Autodesk Fusion 360 part; units mm, degrees
(part 2 of 2)
sketch "Sketch21" plane through (0, 0, 6.5) normal (0, 0, 1) x (-1, 0, 0)
  line L0 (-17.15, -12.5) -> (-13.9, -12.5)
  line L1 (-13.9, -12.5) -> (-13.9, -16.5)
  line L2 (-13.9, -16.5) -> (-17.15, -16.5)
  line L3 (-17.15, -16.5) -> (-17.15, -12.5)
  line L4 (-52.0582, -15.8447) -> (-53.0435, -16.5507)
  line L5 (-53.0435, -16.5507) -> (-52.0582, -17.32)
  line L6 (-52.0582, -17.32) -> (-52.3471, -17.6537)
  line L7 (-52.3471, -17.6537) -> (-53.2, -17)
  line L8 (-53.2, -17) -> (-53.2, -19.1)
  line L9 (-53.2, -19.1) -> (-53.5525, -19.2486)
  line L10 (-53.5525, -19.2486) -> (-55.3569, -17.8655)
  line L11 (-55.3569, -17.8655) -> (-55.3569, -17.6445)
  line L12 (-55.3569, -17.6445) -> (-53.8076, -16.5343)
  line L13 (-53.8076, -16.5343) -> (-55.2956, -15.447)
  line L14 (-55.2956, -15.447) -> (-55.2956, -15.2)
  line L15 (-55.2956, -15.2) -> (-53.5478, -13.8892)
  line L16 (-53.5478, -13.8892) -> (-53.3624, -13.8892)
  line L17 (-53.3624, -13.8892) -> (-53.1862, -14.0561)
  line L18 (-53.1862, -14.0561) -> (-53.1862, -16.0889)
  line L19 (-53.1862, -16.0889) -> (-52.3253, -15.472)
  line L20 (-52.3253, -15.472) -> (-52.0582, -15.8447)
  line L21 (-15.85, -17.05) -> (-15.85, -21.05)
  line L22 (-15.85, -21.05) -> (-19.85, -21.05)
  line L23 (-19.85, -21.05) -> (-19.85, -17.05)
  line L24 (-19.85, -17.05) -> (-15.85, -17.05)
  line L25 (-28.1, -12) -> (-28.1, -6.3)
  line L26 (-28.1, -6.3) -> (-14, -6.3)
  line L27 (-14, -6.3) -> (-14, -12)
  line L28 (-14, -12) -> (-28.1, -12)
  line L29 (-57.9, -11.55) -> (-57.9, -8.9)
  arc A0 (-57.4639, -4.5) -> (-57.9, -8.9) centre (-59.7, -6.5) ccw
  line L30 (-57.4639, -4.5) -> (-46.1, -4.5)
  line L31 (-46.1, -4.5) -> (-46.1, -11.55)
  line L32 (-46.1, -11.55) -> (-57.9, -11.55)
  line L33 (-16.8084, -5.642) -> (-16.8084, -3.2045)
  line L34 (-16.8084, -3.2045) -> (-16.4431, -3.2045)
  line L35 (-16.4431, -3.2045) -> (-16.4431, -6.0678)
  line L36 (-16.4431, -6.0678) -> (-17.0134, -6.0678)
  line L37 (-17.0134, -6.0678) -> (-17.6912, -4.0404)
  spline S0 degree 3 poles (-17.6912, -4.0404) (-17.7185, -3.958) (-17.7651, -3.817) (-17.8095, -3.6754) (-17.8279, -3.6166) knots 0 0 0 0 0.026049 0.044534 0.044534 0.044534 0.044534
  spline S1 degree 3 poles (-17.8279, -3.6166) (-17.8486, -3.6809) (-17.8979, -3.8344) (-17.95, -3.987) (-17.9802, -4.0756) knots 0 0 0 0 0.020274 0.048362 0.048362 0.048362 0.048362
  line L38 (-17.9802, -4.0756) -> (-18.6658, -6.0678)
  line L39 (-18.6658, -6.0678) -> (-19.1756, -6.0678)
  line L40 (-19.1756, -6.0678) -> (-19.1756, -3.2045)
  line L41 (-19.1756, -3.2045) -> (-18.8103, -3.2045)
  line L42 (-18.8103, -3.2045) -> (-18.8103, -5.601)
  line L43 (-18.8103, -5.601) -> (-17.9783, -3.2045)
  line L44 (-17.9783, -3.2045) -> (-17.6365, -3.2045)
  line L45 (-17.6365, -3.2045) -> (-16.8084, -5.642)
  spline S2 degree 3 poles (-27.6951, -3.1556) (-27.5655, -3.1667) (-27.3128, -3.1883) (-27.1326, -3.3659) (-27.0447, -3.4525) knots 0 0 0 0 0.037701 0.073534 0.073534 0.073534 0.073534
  spline S3 degree 3 poles (-27.0447, -3.4525) (-26.9626, -3.606) (-26.7692, -3.9674) (-26.7643, -4.3795) (-26.7615, -4.6166) knots 0 0 0 0 0.051552 0.121345 0.121345 0.121345 0.121345
  spline S4 degree 3 poles (-26.7615, -4.6166) (-26.7636, -4.7702) (-26.7673, -5.047) (-26.8356, -5.3148) (-26.866, -5.434) knots 0 0 0 0 0.0459 0.082658 0.082658 0.082658 0.082658
  spline S5 degree 3 poles (-26.866, -5.434) (-26.903, -5.5295) (-26.9732, -5.7107) (-27.1113, -5.8471) (-27.1765, -5.9115) knots 0 0 0 0 0.030338 0.057541 0.057541 0.057541 0.057541
  spline S6 degree 3 poles (-27.1765, -5.9115) (-27.2518, -5.9605) (-27.4092, -6.0629) (-27.597, -6.0738) (-27.6951, -6.0795) knots 0 0 0 0 0.026458 0.055354 0.055354 0.055354 0.055354
  spline S7 degree 3 poles (-27.6951, -6.0795) (-27.7683, -6.0763) (-27.9088, -6.0701) (-28.0376, -6.0137) (-28.0994, -5.9867) knots 0 0 0 0 0.021755 0.0418 0.0418 0.0418 0.0418
  spline S8 degree 3 poles (-28.0994, -5.9867) (-28.1551, -5.9519) (-28.2681, -5.8814) (-28.3466, -5.7737) (-28.3865, -5.7191) knots 0 0 0 0 0.019498 0.039572 0.039572 0.039572 0.039572
  spline S9 degree 3 poles (-28.3865, -5.7191) (-28.4227, -5.6556) (-28.4995, -5.5211) (-28.5419, -5.372) (-28.5642, -5.2933) knots 0 0 0 0 0.021862 0.046289 0.046289 0.046289 0.046289
  spline S10 degree 3 poles (-28.5642, -5.2933) (-28.583, -5.1954) (-28.6257, -4.972) (-28.6276, -4.7444) (-28.6287, -4.6166) knots 0 0 0 0 0.029862 0.068104 0.068104 0.068104 0.068104
  spline S11 degree 3 poles (-28.6287, -4.6166) (-28.6266, -4.4639) (-28.6228, -4.1886) (-28.5553, -3.9219) (-28.5252, -3.8031) knots 0 0 0 0 0.045606 0.082253 0.082253 0.082253 0.082253
  spline S12 degree 3 poles (-28.5252, -3.8031) (-28.4884, -3.7075) (-28.4186, -3.526) (-28.2808, -3.3893) (-28.2156, -3.3246) knots 0 0 0 0 0.030329 0.05757 0.05757 0.05757 0.05757
  spline S13 degree 3 poles (-28.2156, -3.3246) (-28.1402, -3.2753) (-27.9823, -3.1722) (-27.7937, -3.1613) (-27.6951, -3.1556) knots 0 0 0 0 0.026536 0.05558 0.05558 0.05558 0.05558
  spline S14 degree 3 poles (-24.533, -4.0326) (-24.5377, -4.1203) (-24.5468, -4.2881) (-24.6333, -4.4318) (-24.6746, -4.5004) knots 0 0 0 0 0.025902 0.04954 0.04954 0.04954 0.04954
  spline S15 degree 3 poles (-24.6746, -4.5004) (-24.7283, -4.5586) (-24.8399, -4.6795) (-24.9966, -4.7307) (-25.0779, -4.7572) knots 0 0 0 0 0.023359 0.04853 0.04853 0.04853 0.04853
  spline S16 degree 3 poles (-25.0779, -4.7572) (-25.0111, -4.7849) (-24.8856, -4.8369) (-24.7957, -4.9383) (-24.7537, -4.9857) knots 0 0 0 0 0.021379 0.040128 0.040128 0.040128 0.040128
  spline S17 degree 3 poles (-24.7537, -4.9857) (-24.7229, -5.0388) (-24.6592, -5.1486) (-24.652, -5.2755) (-24.6482, -5.3412) knots 0 0 0 0 0.018126 0.037544 0.037544 0.037544 0.037544
  spline S18 degree 3 poles (-24.6482, -5.3412) (-24.6575, -5.4411) (-24.6759, -5.6404) (-24.8073, -5.7913) (-24.8728, -5.8666) knots 0 0 0 0 0.029303 0.058444 0.058444 0.058444 0.058444
  spline S19 degree 3 poles (-24.8728, -5.8666) (-24.9568, -5.9286) (-25.134, -6.0595) (-25.3545, -6.0726) (-25.4705, -6.0795) knots 0 0 0 0 0.030658 0.064671 0.064671 0.064671 0.064671
  spline S20 degree 3 poles (-25.4705, -6.0795) (-25.5873, -6.0723) (-25.8104, -6.0585) (-25.989, -5.9252) (-26.074, -5.8617) knots 0 0 0 0 0.034273 0.065414 0.065414 0.065414 0.065414
  spline S21 degree 3 poles (-26.074, -5.8617) (-26.1406, -5.7853) (-26.2736, -5.633) (-26.2929, -5.4317) (-26.3025, -5.3314) knots 0 0 0 0 0.02961 0.059051 0.059051 0.059051 0.059051
  spline S22 degree 3 poles (-26.3025, -5.3314) (-26.2986, -5.2679) (-26.2911, -5.144) (-26.2285, -5.0369) (-26.198, -4.9847) knots 0 0 0 0 0.01881 0.036662 0.036662 0.036662 0.036662
  spline S23 degree 3 poles (-26.198, -4.9847) (-26.1567, -4.9377) (-26.0687, -4.8375) (-25.9458, -4.785) (-25.8806, -4.7572) knots 0 0 0 0 0.018541 0.039496 0.039496 0.039496 0.039496
  spline S24 degree 3 poles (-25.8806, -4.7572) (-25.9622, -4.7257) (-26.1184, -4.6652) (-26.2291, -4.5398) (-26.282, -4.4799) knots 0 0 0 0 0.025791 0.049427 0.049427 0.049427 0.049427
  spline S25 degree 3 poles (-26.282, -4.4799) (-26.3222, -4.4116) (-26.4051, -4.2707) (-26.4147, -4.1072) (-26.4197, -4.0228) knots 0 0 0 0 0.023398 0.048344 0.048344 0.048344 0.048344
  spline S26 degree 3 poles (-26.4197, -4.0228) (-26.4091, -3.9055) (-26.388, -3.6722) (-26.2357, -3.4942) (-26.1599, -3.4056) knots 0 0 0 0 0.034407 0.068461 0.068461 0.068461 0.068461
  spline S27 degree 3 poles (-26.1599, -3.4056) (-26.0636, -3.3328) (-25.8618, -3.1801) (-25.6086, -3.164) (-25.4763, -3.1556) knots 0 0 0 0 0.035444 0.074232 0.074232 0.074232 0.074232
  spline S28 degree 3 poles (-25.4763, -3.1556) (-25.344, -3.1641) (-25.0907, -3.1803) (-24.8891, -3.3335) (-24.7927, -3.4066) knots 0 0 0 0 0.038792 0.074275 0.074275 0.074275 0.074275
  spline S29 degree 3 poles (-24.7927, -3.4066) (-24.717, -3.4961) (-24.5638, -3.677) (-24.5433, -3.9132) (-24.533, -4.0326) knots 0 0 0 0 0.034274 0.069281 0.069281 0.069281 0.069281
  line L46 (-61.2402, -13.1835) -> (-61.2402, -11.8827)
  line L47 (-61.2402, -11.8827) -> (-60.8613, -11.8827)
  line L48 (-60.8613, -11.8827) -> (-60.8613, -14.746)
  line L49 (-60.8613, -14.746) -> (-62.793, -14.746)
  line L50 (-62.793, -14.746) -> (-62.793, -14.4081)
  line L51 (-62.793, -14.4081) -> (-61.2402, -14.4081)
  line L52 (-61.2402, -14.4081) -> (-61.2402, -13.5213)
  line L53 (-61.2402, -13.5213) -> (-62.584, -13.5213)
  line L54 (-62.584, -13.5213) -> (-62.584, -13.1835)
  line L55 (-62.584, -13.1835) -> (-61.2402, -13.1835)
  line L56 (-50.1317, -14.1836) -> (-50.1317, -11.9336)
  line L57 (-50.1317, -11.9336) -> (-49.7684, -11.9336)
  line L58 (-49.7684, -11.9336) -> (-49.7684, -14.7969)
  line L59 (-49.7684, -14.7969) -> (-50.1571, -14.7969)
  line L60 (-50.1571, -14.7969) -> (-51.661, -12.5488)
  line L61 (-51.661, -12.5488) -> (-51.661, -14.7969)
  line L62 (-51.661, -14.7969) -> (-52.0243, -14.7969)
  line L63 (-52.0243, -14.7969) -> (-52.0243, -11.9336)
  line L64 (-52.0243, -11.9336) -> (-51.6356, -11.9336)
  line L65 (-51.6356, -11.9336) -> (-50.1317, -14.1836)
  spline S30 degree 3 poles (-47.1923, -12.0801) (-47.0925, -12.1512) (-46.8928, -12.2937) (-46.7709, -12.5067) (-46.7098, -12.6133) knots 0 0 0 0 0.03628 0.072668 0.072668 0.072668 0.072668
  spline S31 degree 3 poles (-46.7098, -12.6133) (-46.662, -12.7276) (-46.5662, -12.9565) (-46.5526, -13.2042) (-46.5458, -13.3281) knots 0 0 0 0 0.036879 0.073826 0.073826 0.073826 0.073826
  spline S32 degree 3 poles (-46.5458, -13.3281) (-46.5569, -13.5474) (-46.5776, -13.9578) (-46.8171, -14.2898) (-46.9286, -14.4444) knots 0 0 0 0 0.064266 0.120259 0.120259 0.120259 0.120259
  spline S33 degree 3 poles (-46.9286, -14.4444) (-47.0678, -14.562) (-47.3531, -14.803) (-47.726, -14.8325) (-47.9169, -14.8477) knots 0 0 0 0 0.053269 0.109167 0.109167 0.109167 0.109167
  spline S34 degree 3 poles (-47.9169, -14.8477) (-48.0448, -14.8404) (-48.2961, -14.826) (-48.5212, -14.7135) (-48.6317, -14.6582) knots 0 0 0 0 0.037992 0.074647 0.074647 0.074647 0.074647
  spline S35 degree 3 poles (-48.6317, -14.6582) (-48.7317, -14.5886) (-48.9326, -14.4485) (-49.0554, -14.2365) (-49.1171, -14.1299) knots 0 0 0 0 0.036074 0.072525 0.072525 0.072525 0.072525
  spline S36 degree 3 poles (-49.1171, -14.1299) (-49.1658, -14.0109) (-49.2665, -13.7647) (-49.2781, -13.4988) (-49.2841, -13.3613) knots 0 0 0 0 0.038265 0.079177 0.079177 0.079177 0.079177
  spline S37 degree 3 poles (-49.2841, -13.3613) (-49.2777, -13.2219) (-49.2654, -12.9515) (-49.1595, -12.7026) (-49.1083, -12.582) knots 0 0 0 0 0.041493 0.080461 0.080461 0.080461 0.080461
  spline S38 degree 3 poles (-49.1083, -12.582) (-49.0443, -12.4748) (-48.918, -12.2632) (-48.7119, -12.1282) (-48.6102, -12.0615) knots 0 0 0 0 0.036922 0.072885 0.072885 0.072885 0.072885
  spline S39 degree 3 poles (-48.6102, -12.0615) (-48.5005, -12.01) (-48.28, -11.9065) (-48.0369, -11.892) (-47.9149, -11.8848) knots 0 0 0 0 0.036024 0.072329 0.072329 0.072329 0.072329
  spline S40 degree 3 poles (-47.9149, -11.8848) (-47.7849, -11.8922) (-47.5302, -11.9068) (-47.3033, -12.0231) (-47.1923, -12.0801) knots 0 0 0 0 0.038591 0.075598 0.075598 0.075598 0.075598
  line L66 (-58.7969, -13.1835) -> (-58.7969, -11.8827)
  line L67 (-58.7969, -11.8827) -> (-58.418, -11.8827)
  line L68 (-58.418, -11.8827) -> (-58.418, -14.746)
  line L69 (-58.418, -14.746) -> (-60.3496, -14.746)
  line L70 (-60.3496, -14.746) -> (-60.3496, -14.4081)
  line L71 (-60.3496, -14.4081) -> (-58.7969, -14.4081)
  line L72 (-58.7969, -14.4081) -> (-58.7969, -13.5213)
  line L73 (-58.7969, -13.5213) -> (-60.1406, -13.5213)
  line L74 (-60.1406, -13.5213) -> (-60.1406, -13.1835)
  line L75 (-60.1406, -13.1835) -> (-58.7969, -13.1835)
  spline S41 degree 3 poles (-55.8183, -12.0292) (-55.7186, -12.1003) (-55.5188, -12.2428) (-55.397, -12.4557) (-55.3359, -12.5624) knots 0 0 0 0 0.03628 0.072668 0.072668 0.072668 0.072668
  spline S42 degree 3 poles (-55.3359, -12.5624) (-55.2881, -12.6767) (-55.1923, -12.9055) (-55.1787, -13.1532) (-55.1719, -13.2772) knots 0 0 0 0 0.036879 0.073826 0.073826 0.073826 0.073826
  spline S43 degree 3 poles (-55.1719, -13.2772) (-55.1829, -13.4965) (-55.2037, -13.9068) (-55.4432, -14.2388) (-55.5547, -14.3934) knots 0 0 0 0 0.064266 0.120259 0.120259 0.120259 0.120259
  spline S44 degree 3 poles (-55.5547, -14.3934) (-55.6939, -14.511) (-55.9792, -14.7521) (-56.352, -14.7816) (-56.543, -14.7967) knots 0 0 0 0 0.053269 0.109167 0.109167 0.109167 0.109167
  spline S45 degree 3 poles (-56.543, -14.7967) (-56.6709, -14.7894) (-56.9222, -14.7751) (-57.1473, -14.6625) (-57.2578, -14.6073) knots 0 0 0 0 0.037992 0.074647 0.074647 0.074647 0.074647
  spline S46 degree 3 poles (-57.2578, -14.6073) (-57.3578, -14.5376) (-57.5587, -14.3975) (-57.6815, -14.1855) (-57.7431, -14.079) knots 0 0 0 0 0.036074 0.072525 0.072525 0.072525 0.072525
  spline S47 degree 3 poles (-57.7431, -14.079) (-57.7918, -13.96) (-57.8926, -13.7138) (-57.9042, -13.4478) (-57.9101, -13.3104) knots 0 0 0 0 0.038265 0.079177 0.079177 0.079177 0.079177
  spline S48 degree 3 poles (-57.9101, -13.3104) (-57.9038, -13.171) (-57.8914, -12.9006) (-57.7856, -12.6517) (-57.7344, -12.5311) knots 0 0 0 0 0.041493 0.080461 0.080461 0.080461 0.080461
  spline S49 degree 3 poles (-57.7344, -12.5311) (-57.6704, -12.4239) (-57.5441, -12.2122) (-57.338, -12.0772) (-57.2363, -12.0106) knots 0 0 0 0 0.036922 0.072885 0.072885 0.072885 0.072885
  spline S50 degree 3 poles (-57.2363, -12.0106) (-57.1265, -11.959) (-56.9061, -11.8555) (-56.663, -11.8411) (-56.541, -11.8338) knots 0 0 0 0 0.036024 0.072329 0.072329 0.072329 0.072329
  spline S51 degree 3 poles (-56.541, -11.8338) (-56.411, -11.8413) (-56.1563, -11.8558) (-55.9294, -11.9722) (-55.8183, -12.0292) knots 0 0 0 0 0.038591 0.075598 0.075598 0.075598 0.075598
  spline S52 degree 3 poles (-22.9041, -3.7328) (-22.8758, -3.7018) (-22.8214, -3.6422) (-22.777, -3.5748) (-22.7556, -3.5424) knots 0 0 0 0 0.012549 0.024178 0.024178 0.024178 0.024178
  line L76 (-22.7556, -3.5424) -> (-24.1599, -3.5424)
  line L77 (-24.1599, -3.5424) -> (-24.1599, -3.2045)
  line L78 (-24.1599, -3.2045) -> (-22.2674, -3.2045)
  spline S53 degree 3 poles (-22.2674, -3.2045) (-22.2681, -3.2463) (-22.2695, -3.3298) (-22.2954, -3.4091) (-22.3084, -3.4486) knots 0 0 0 0 0.012479 0.024881 0.024881 0.024881 0.024881
  spline S54 degree 3 poles (-22.3084, -3.4486) (-22.3372, -3.5141) (-22.3975, -3.6512) (-22.491, -3.7683) (-22.5398, -3.8295) knots 0 0 0 0 0.021368 0.044735 0.044735 0.044735 0.044735
  spline S55 degree 3 poles (-22.5398, -3.8295) (-22.6034, -3.8982) (-22.7469, -4.0531) (-22.9094, -4.188) (-22.9998, -4.2631) knots 0 0 0 0 0.028058 0.063271 0.063271 0.063271 0.063271
  spline S56 degree 3 poles (-22.9998, -4.2631) (-23.1342, -4.3733) (-23.3607, -4.5589) (-23.5526, -4.7798) (-23.6306, -4.8695) knots 0 0 0 0 0.052022 0.087641 0.087641 0.087641 0.087641
  spline S57 degree 3 poles (-23.6306, -4.8695) (-23.6784, -4.9395) (-23.7661, -5.0682) (-23.7857, -5.2222) (-23.7947, -5.2924) knots 0 0 0 0 0.024992 0.04593 0.04593 0.04593 0.04593
  spline S58 degree 3 poles (-23.7947, -5.2924) (-23.7885, -5.3592) (-23.7762, -5.4927) (-23.6889, -5.5942) (-23.6453, -5.6449) knots 0 0 0 0 0.019622 0.039148 0.039148 0.039148 0.039148
  spline S59 degree 3 poles (-23.6453, -5.6449) (-23.5902, -5.6868) (-23.4752, -5.774) (-23.3308, -5.7835) (-23.2556, -5.7885) knots 0 0 0 0 0.020302 0.042349 0.042349 0.042349 0.042349
  spline S60 degree 3 poles (-23.2556, -5.7885) (-23.1765, -5.7834) (-23.0253, -5.7736) (-22.9062, -5.6805) (-22.8494, -5.6361) knots 0 0 0 0 0.023167 0.044296 0.044296 0.044296 0.044296
  spline S61 degree 3 poles (-22.8494, -5.6361) (-22.8049, -5.5779) (-22.71, -5.4538) (-22.7003, -5.2974) (-22.6951, -5.2142) knots 0 0 0 0 0.021485 0.045832 0.045832 0.045832 0.045832
  line L79 (-22.6951, -5.2142) -> (-22.3338, -5.2513)
  spline S62 degree 3 poles (-22.3338, -5.2513) (-22.3518, -5.3754) (-22.3857, -5.6086) (-22.5406, -5.785) (-22.6131, -5.8676) knots 0 0 0 0 0.0367 0.068958 0.068958 0.068958 0.068958
  spline S63 degree 3 poles (-22.6131, -5.8676) (-22.7047, -5.9293) (-22.9006, -6.0614) (-23.1374, -6.0732) (-23.2634, -6.0795) knots 0 0 0 0 0.032518 0.069569 0.069569 0.069569 0.069569
  spline S64 degree 3 poles (-23.2634, -6.0795) (-23.3909, -6.0725) (-23.6312, -6.0593) (-23.8248, -5.9175) (-23.9158, -5.851) knots 0 0 0 0 0.037354 0.070456 0.070456 0.070456 0.070456
  spline S65 degree 3 poles (-23.9158, -5.851) (-23.9859, -5.7699) (-24.1267, -5.607) (-24.1462, -5.3924) (-24.156, -5.2845) knots 0 0 0 0 0.031293 0.062923 0.062923 0.062923 0.062923
  spline S66 degree 3 poles (-24.156, -5.2845) (-24.153, -5.2272) (-24.1467, -5.111) (-24.1062, -5.0019) (-24.0857, -4.9467) knots 0 0 0 0 0.017131 0.03469 0.03469 0.03469 0.03469
  spline S67 degree 3 poles (-24.0857, -4.9467) (-24.0566, -4.8885) (-23.9933, -4.7624) (-23.9017, -4.655) (-23.8523, -4.597) knots 0 0 0 0 0.019438 0.042172 0.042172 0.042172 0.042172
  spline S68 degree 3 poles (-23.8523, -4.597) (-23.7809, -4.5234) (-23.609, -4.3462) (-23.4205, -4.1865) (-23.3103, -4.0931) knots 0 0 0 0 0.030746 0.074043 0.074043 0.074043 0.074043
  spline S69 degree 3 poles (-23.3103, -4.0931) (-23.2227, -4.02) (-23.0836, -3.904) (-22.9525, -3.779) (-22.9041, -3.7328) knots 0 0 0 0 0.034229 0.054317 0.054317 0.054317 0.054317
  line L80 (-20.1658, -4.3685) -> (-20.1658, -3.2045)
  line L81 (-20.1658, -3.2045) -> (-19.7869, -3.2045)
  line L82 (-19.7869, -3.2045) -> (-19.7869, -6.0678)
  line L83 (-19.7869, -6.0678) -> (-20.867, -6.0678)
  spline S70 degree 3 poles (-20.867, -6.0678) (-20.9509, -6.0675) (-21.0967, -6.067) (-21.2412, -6.0483) (-21.3025, -6.0404) knots 0 0 0 0 0.025156 0.043678 0.043678 0.043678 0.043678
  spline S71 degree 3 poles (-21.3025, -6.0404) (-21.3685, -6.027) (-21.4938, -6.0016) (-21.6039, -5.9371) (-21.656, -5.9066) knots 0 0 0 0 0.020045 0.038029 0.038029 0.038029 0.038029
  spline S72 degree 3 poles (-21.656, -5.9066) (-21.7017, -5.8695) (-21.7963, -5.7925) (-21.8551, -5.6856) (-21.8855, -5.6303) knots 0 0 0 0 0.017485 0.036225 0.036225 0.036225 0.036225
  spline S73 degree 3 poles (-21.8855, -5.6303) (-21.9109, -5.5689) (-21.9625, -5.4438) (-21.9691, -5.3085) (-21.9724, -5.2396) knots 0 0 0 0 0.019759 0.040284 0.040284 0.040284 0.040284
  spline S74 degree 3 poles (-21.9724, -5.2396) (-21.9634, -5.1233) (-21.9457, -4.8946) (-21.8078, -4.7115) (-21.74, -4.6215) knots 0 0 0 0 0.034213 0.067281 0.067281 0.067281 0.067281
  spline S75 degree 3 poles (-21.74, -4.6215) (-21.6347, -4.5481) (-21.3849, -4.3742) (-21.0778, -4.3706) (-20.9002, -4.3685) knots 0 0 0 0 0.037732 0.089487 0.089487 0.089487 0.089487
  line L84 (-20.9002, -4.3685) -> (-20.1658, -4.3685)
  spline S76 degree 3 poles (-15.325, -3.2523) (-15.2553, -3.2384) (-15.1029, -3.2079) (-14.9474, -3.2057) (-14.8631, -3.2045) knots 0 0 0 0 0.021277 0.046525 0.046525 0.046525 0.046525
  line L85 (-14.8631, -3.2045) -> (-13.7713, -3.2045)
  line L86 (-13.7713, -3.2045) -> (-13.7713, -6.0678)
  line L87 (-13.7713, -6.0678) -> (-14.8455, -6.0678)
  spline S77 degree 3 poles (-14.8455, -6.0678) (-14.945, -6.0659) (-15.125, -6.0626) (-15.2956, -6.0061) (-15.3718, -5.9808) knots 0 0 0 0 0.029645 0.05362 0.05362 0.05362 0.05362
  spline S78 degree 3 poles (-15.3718, -5.9808) (-15.4343, -5.9481) (-15.5585, -5.8829) (-15.6412, -5.7696) (-15.6824, -5.7133) knots 0 0 0 0 0.020838 0.041482 0.041482 0.041482 0.041482
  spline S79 degree 3 poles (-15.6824, -5.7133) (-15.7151, -5.653) (-15.7794, -5.5349) (-15.7897, -5.401) (-15.7947, -5.3353) knots 0 0 0 0 0.02031 0.039825 0.039825 0.039825 0.039825
  spline S80 degree 3 poles (-15.7947, -5.3353) (-15.7904, -5.2748) (-15.7817, -5.1525) (-15.7241, -5.0443) (-15.6951, -4.9896) knots 0 0 0 0 0.017995 0.036334 0.036334 0.036334 0.036334
  spline S81 degree 3 poles (-15.6951, -4.9896) (-15.6563, -4.9375) (-15.5752, -4.8286) (-15.4563, -4.7624) (-15.3943, -4.7279) knots 0 0 0 0 0.019257 0.040275 0.040275 0.040275 0.040275
  spline S82 degree 3 poles (-15.3943, -4.7279) (-15.4748, -4.6995) (-15.6291, -4.6449) (-15.7404, -4.5253) (-15.7937, -4.4681) knots 0 0 0 0 0.025178 0.048277 0.048277 0.048277 0.048277
  spline S83 degree 3 poles (-15.7937, -4.4681) (-15.8344, -4.4033) (-15.9177, -4.2707) (-15.9281, -4.1144) (-15.9334, -4.0345) knots 0 0 0 0 0.022594 0.046193 0.046193 0.046193 0.046193
  spline S84 degree 3 poles (-15.9334, -4.0345) (-15.93, -3.969) (-15.9233, -3.8394) (-15.8732, -3.7197) (-15.8484, -3.6605) knots 0 0 0 0 0.019525 0.038613 0.038613 0.038613 0.038613
  spline S85 degree 3 poles (-15.8484, -3.6605) (-15.8197, -3.6072) (-15.7652, -3.506) (-15.6791, -3.4299) (-15.6384, -3.3939) knots 0 0 0 0 0.018014 0.034173 0.034173 0.034173 0.034173
  spline S86 degree 3 poles (-15.6384, -3.3939) (-15.5925, -3.3642) (-15.4953, -3.3012) (-15.3838, -3.2692) (-15.325, -3.2523) knots 0 0 0 0 0.016314 0.034565 0.034565 0.034565 0.034565
  line L88 (-44, -14.3465) -> (-44, -8.4135)
  arc A1 (-44, -14.3465) -> (-44, -8.4135) centre (-38.9, -11.38) ccw
  circle A2 centre (-9.7, -18.5) radius 3
  circle A3 centre (-59.7, -18.5) radius 3
  line L89 (-3, -22) -> (-3, -3)
  line L90 (-3, -3) -> (-66.4, -3)
  line L91 (-66.4, -3) -> (-66.4, -22)
  line L92 (-66.4, -22) -> (-3, -22)
  circle A4 centre (-9.7, -6.5) radius 3
  circle A5 centre (-38.9, -11.38) radius 7.9
  line L93 (-56.4, -6) -> (-47.6, -6)
  line L94 (-47.6, -6) -> (-47.6, -10.05)
  line L95 (-47.6, -10.05) -> (-56.4, -10.05)
  line L96 (-56.4, -10.05) -> (-56.4, -6)
  line L97 (-57.9, -11.55) -> (-46.1, -11.55)
  line L98 (-46.1, -11.55) -> (-46.1, -4.5)
  line L99 (-46.1, -4.5) -> (-57.9, -4.5)
  line L100 (-57.9, -4.5) -> (-57.9, -11.55)
  dimension "d162" = 15.8
  constraint concentric A1 A5
  measures "d162" diameter of A5
extrude "Extrude25" cut sketch "Sketch21" against normal up to surface (4.5 mm away) contours L31 L32 A5 L97 L98 bodies 1
sketch "Sketch13" plane through (0, 0, 2) normal (0, 0, 1) x (-1, 0, 0)
  spline S0 degree 5 poles (-13, -21) (-12.9646, -20.9538) (-12.9119, -20.8347) (-12.8858, -20.5685) (-12.9434, -20.0302) (-13.1125, -19.1087) (-13.3117, -18.0419) (-13.4771, -16.9472) (-13.5596, -15.9266) (-13.5404, -15.0289) (-13.4343, -14.2416) (-13.2755, -13.5173) (-13.1092, -12.792) (-12.9804, -12.0068) (-12.9236, -11.1274) (-12.9529, -10.1651) (-13.0679, -9.1622) (-13.2599, -8.1778) (-13.5174, -7.2746) (-13.8326, -6.5044) (-14.2066, -5.8947) (-14.6566, -5.4341) (-15.207, -5.0857) (-15.8804, -4.8045) (-16.6894, -4.551) (-17.6257, -4.3096) (-18.6571, -4.0958) (-19.7378, -3.9412) (-20.8164, -3.8828) (-21.8447, -3.951) (-22.787, -4.1576) (-23.627, -4.4852) (-24.3799, -4.8712) (-25.083, -5.2256) (-25.7801, -5.4598) (-26.5066, -5.5143) (-27.2774, -5.3814) (-28.0674, -5.1423) (-28.8173, -4.9489) (-29.4603, -4.9571) (-29.9425, -5.2749) (-30.2462, -5.903) (-30.411, -6.6831) (-30.5087, -7.3832) (-30.6209, -7.7798) (-30.8155, -7.7387) (-31.1224, -7.3008) (-31.5439, -6.6155) (-32.0647, -5.8711) (-32.6632, -5.2226) (-33.3205, -4.7328) (-34.0208, -4.4037) (-34.7521, -4.1964) (-35.5076, -4.0563) (-36.2858, -3.9352) (-37.0922, -3.816) (-37.9338, -3.7038) (-38.8151, -3.6163) (-39.7321, -3.5743) (-40.6685, -3.5925) (-41.5893, -3.6694) (-42.4405, -3.7812) (-43.1695, -3.8957) (-43.7428, -3.9816) (-44.162, -4.0192) (-44.4879, -4.0139) (-44.8361, -3.9961) (-45.3251, -3.9983) (-46.0262, -4.0325) (-46.9576, -4.09) (-48.1, -4.1501) (-49.4051, -4.1861) (-50.807, -4.1726) (-52.2321, -4.0922) (-53.6096, -3.942) (-54.8832, -3.7418) (-56.0162, -3.5346) (-56.9873, -3.374) (-57.7887, -3.3164) (-58.4239, -3.4101) (-58.905, -3.6869) (-59.25, -4.1503) (-59.4811, -4.7715) (-59.6226, -5.5047) (-59.6985, -6.3001) (-59.7314, -7.117) (-59.74, -7.9395) (-59.738, -8.7698) (-59.7325, -9.6146) (-59.7232, -10.4729) (-59.7008, -11.3245) (-59.6455, -12.1155) (-59.5272, -12.7538) (-59.3147, -13.1527) (-58.9833, -13.2631) (-58.524, -13.1203) (-57.9462, -12.8479) (-57.2688, -12.5953) (-56.5149, -12.4963) (-55.703, -12.6088) (-54.845, -12.8988) (-53.9498, -13.2806) (-53.0259, -13.6426) (-52.084, -13.8807) (-51.14, -13.9251) (-50.2184, -13.777) (-49.3515, -13.516) (-48.5715, -13.2601) (-47.9036, -13.1361) (-47.3594, -13.2479) (-46.9292, -13.6421) (-46.5776, -14.284) (-46.2552, -15.0899) (-45.9094, -15.9514) (-45.4942, -16.7625) (-44.9816, -17.4463) (-44.3712, -17.9808) (-43.6815, -18.3816) (-42.9411, -18.6874) (-42.18, -18.9436) (-41.4217, -19.1877) (-40.6728, -19.4311) (-39.9263, -19.6627) (-39.1696, -19.8587) (-38.3905, -19.9908) (-37.5836, -20.0344) (-36.7581, -19.9781) (-35.938, -19.8256) (-35.1537, -19.5879) (-34.4364, -19.278) (-33.8113, -18.9061) (-33.2903, -18.4721) (-32.8689, -17.9643) (-32.5302, -17.3706) (-32.2496, -16.6882) (-31.9981, -15.9329) (-31.7469, -15.1513) (-31.47, -14.4118) (-31.1455, -13.7851) (-30.7582, -13.3272) (-30.3011, -13.0632) (-29.7777, -12.9676) (-29.1964, -12.9837) (-28.5638, -13.0466) (-27.8775, -13.1062) (-27.122, -13.1459) (-26.2779, -13.1708) (-25.3307, -13.1998) (-24.2794, -13.2565) (-23.1447, -13.3606) (-21.9789, -13.5181) (-20.8692, -13.7162) (-19.9163, -13.9348) (-19.2194, -14.1535) (-18.8571, -14.362) (-18.8728, -14.5665) (-19.2525, -14.8023) (-19.9322, -15.1233) (-20.8154, -15.583) (-21.7869, -16.2177) (-22.7283, -17.0314) (-23.534, -17.9737) (-24.1189, -18.9515) (-24.4213, -19.8556) (-24.4084, -20.5827) (-24.0797, -21.0596) (-23.4718, -21.2655) (-22.6629, -21.2565) (-21.7532, -21.1343) (-20.8453, -21.0145) (-20.0236, -20.9936) (-19.3364, -21.1204) (-18.7706, -21.3549) (-18.2675, -21.5959) (-17.7548, -21.7362) (-17.1708, -21.7036) (-16.498, -21.5205) (-15.7591, -21.2787) (-15.0018, -21.0851) (-14.2874, -21.0186) (-13.6777, -21.0811) (-13.3139, -21.1384) (-13.1244, -21.1121) (-13.0354, -21.0462) (-13, -21) knots 0 0 0 0 0 0 0.00555556 0.01111111 0.01666667 0.02222222 0.02777778 0.03333333 0.03888889 0.04444444 0.05 0.05555556 0.06111111 0.06666667 0.07222222 0.07777778 0.08333333 0.08888889 0.09444444 0.1 0.10555556 0.11111111 0.11666667 0.12222222 0.12777778 0.13333333 0.13888889 0.14444444 0.15 0.15555556 0.16111111 0.16666667 0.17222222 0.17777778 0.18333333 0.18888889 0.19444444 0.2 0.20555556 0.21111111 0.21666667 0.22222222 0.22777778 0.23333333 0.23888889 0.24444444 0.25 0.25555556 0.26111111 0.26666667 0.27222222 0.27777778 0.28333333 0.28888889 0.29444444 0.3 0.30555556 0.31111111 0.31666667 0.32222222 0.32777778 0.33333333 0.33888889 0.34444444 0.35 0.35555556 0.36111111 0.36666667 0.37222222 0.37777778 0.38333333 0.38888889 0.39444444 0.4 0.40555556 0.41111111 0.41666667 0.42222222 0.42777778 0.43333333 0.43888889 0.44444444 0.45 0.45555556 0.46111111 0.46666667 0.47222222 0.47777778 0.48333333 0.48888889 0.49444444 0.5 0.50555556 0.51111111 0.51666667 0.52222222 0.52777778 0.53333333 0.53888889 0.54444444 0.55 0.55555556 0.56111111 0.56666667 0.57222222 0.57777778 0.58333333 0.58888889 0.59444444 0.6 0.60555556 0.61111111 0.61666667 0.62222222 0.62777778 0.63333333 0.63888889 0.64444444 0.65 0.65555556 0.66111111 0.66666667 0.67222222 0.67777778 0.68333333 0.68888889 0.69444444 0.7 0.70555556 0.71111111 0.71666667 0.72222222 0.72777778 0.73333333 0.73888889 0.74444444 0.75 0.75555556 0.76111111 0.76666667 0.77222222 0.77777778 0.78333333 0.78888889 0.79444444 0.8 0.80555556 0.81111111 0.81666667 0.82222222 0.82777778 0.83333333 0.83888889 0.84444444 0.85 0.85555556 0.86111111 0.86666667 0.87222222 0.87777778 0.88333333 0.88888889 0.89444444 0.9 0.90555556 0.91111111 0.91666667 0.92222222 0.92777778 0.93333333 0.93888889 0.94444444 0.95 0.95555556 0.96111111 0.96666667 0.97222222 0.97777778 0.98333333 0.98888889 0.99444444 1 1 1 1 1 1
  spline S1 degree 3 poles (-27.6912, -5.7885) (-27.6143, -5.7796) (-27.4588, -5.7616) (-27.3563, -5.6432) (-27.3045, -5.5834) knots 0 0 0 0 0.022373 0.04522 0.04522 0.04522 0.04522
  spline S2 degree 3 poles (-27.3045, -5.5834) (-27.252, -5.4607) (-27.1207, -5.1538) (-27.122, -4.8181) (-27.1228, -4.6166) knots 0 0 0 0 0.039668 0.099266 0.099266 0.099266 0.099266
  spline S3 degree 3 poles (-27.1228, -4.6166) (-27.1208, -4.4176) (-27.1176, -4.0927) (-27.2403, -3.7939) (-27.2879, -3.6781) knots 0 0 0 0 0.058861 0.096109 0.096109 0.096109 0.096109
  spline S4 degree 3 poles (-27.2879, -3.6781) (-27.3439, -3.6101) (-27.4508, -3.4804) (-27.6164, -3.4562) (-27.6951, -3.4447) knots 0 0 0 0 0.02542 0.048461 0.048461 0.048461 0.048461
  spline S5 degree 3 poles (-27.6951, -3.4447) (-27.7738, -3.4563) (-27.9396, -3.4807) (-28.0463, -3.6108) (-28.1023, -3.6791) knots 0 0 0 0 0.023047 0.048518 0.048518 0.048518 0.048518
  spline S6 degree 3 poles (-28.1023, -3.6791) (-28.1499, -3.795) (-28.2724, -4.0935) (-28.2693, -4.418) (-28.2674, -4.6166) knots 0 0 0 0 0.037272 0.09601 0.09601 0.09601 0.09601
  spline S7 degree 3 poles (-28.2674, -4.6166) (-28.2694, -4.816) (-28.2728, -5.1412) (-28.1499, -5.4403) (-28.1023, -5.556) knots 0 0 0 0 0.058982 0.096208 0.096208 0.096208 0.096208
  spline S8 degree 3 poles (-28.1023, -5.556) (-28.0459, -5.6238) (-27.9377, -5.7536) (-27.7709, -5.7772) (-27.6912, -5.7885) knots 0 0 0 0 0.025441 0.048759 0.048759 0.048759 0.048759
  line L0 (-54.6684, -16.0889) -> (-54.6684, -14.5476)
  line L1 (-54.6684, -14.5476) -> (-55.7, -15.3)
  line L2 (-55.7, -15.3) -> (-54.6684, -16.0889)
  line L3 (-55.7374, -17.7798) -> (-54.6684, -18.5974)
  line L4 (-54.6684, -18.5974) -> (-54.6684, -17.0001)
  line L5 (-54.6684, -17.0001) -> (-55.7374, -17.7798)
  line L6 (-14.8123, -4.5267) -> (-14.1502, -4.5267)
  line L7 (-14.1502, -4.5267) -> (-14.1502, -3.5424)
  line L8 (-14.1502, -3.5424) -> (-14.8631, -3.5424)
  spline S9 degree 3 poles (-14.8631, -3.5424) (-14.9152, -3.5423) (-15.0014, -3.5421) (-15.087, -3.5521) (-15.1209, -3.556) knots 0 0 0 0 0.015629 0.025837 0.025837 0.025837 0.025837
  spline S10 degree 3 poles (-15.1209, -3.556) (-15.1616, -3.5645) (-15.2382, -3.5804) (-15.3073, -3.617) (-15.3396, -3.6342) knots 0 0 0 0 0.012412 0.023332 0.023332 0.023332 0.023332
  spline S11 degree 3 poles (-15.3396, -3.6342) (-15.3679, -3.6551) (-15.4267, -3.6984) (-15.4645, -3.7609) (-15.4842, -3.7933) knots 0 0 0 0 0.01045 0.021686 0.021686 0.021686 0.021686
  spline S12 degree 3 poles (-15.4842, -3.7933) (-15.5007, -3.8303) (-15.5349, -3.907) (-15.5388, -3.991) (-15.5408, -4.0345) knots 0 0 0 0 0.01203 0.024974 0.024974 0.024974 0.024974
  spline S13 degree 3 poles (-15.5408, -4.0345) (-15.5378, -4.0856) (-15.5319, -4.1848) (-15.4827, -4.271) (-15.4588, -4.3129) knots 0 0 0 0 0.015106 0.029367 0.029367 0.029367 0.029367
  spline S14 degree 3 poles (-15.4588, -4.3129) (-15.4284, -4.3495) (-15.3665, -4.4239) (-15.2768, -4.4603) (-15.2312, -4.4789) knots 0 0 0 0 0.014036 0.028558 0.028558 0.028558 0.028558
  spline S15 degree 3 poles (-15.2312, -4.4789) (-15.1723, -4.4928) (-15.0347, -4.5252) (-14.8932, -4.5262) (-14.8123, -4.5267) knots 0 0 0 0 0.018108 0.042283 0.042283 0.042283 0.042283
  line L9 (-14.7224, -5.7299) -> (-14.1502, -5.7299)
  line L10 (-14.1502, -5.7299) -> (-14.1502, -4.8646)
  line L11 (-14.1502, -4.8646) -> (-14.7693, -4.8646)
  spline S16 degree 3 poles (-14.7693, -4.8646) (-14.8417, -4.8646) (-14.9633, -4.8645) (-15.0824, -4.8882) (-15.1306, -4.8978) knots 0 0 0 0 0.021647 0.036361 0.036361 0.036361 0.036361
  spline S17 degree 3 poles (-15.1306, -4.8978) (-15.1751, -4.9135) (-15.2595, -4.9434) (-15.3199, -5.0092) (-15.3484, -5.0404) knots 0 0 0 0 0.013899 0.026387 0.026387 0.026387 0.026387
  spline S18 degree 3 poles (-15.3484, -5.0404) (-15.3698, -5.0769) (-15.4148, -5.154) (-15.4193, -5.2434) (-15.4217, -5.2904) knots 0 0 0 0 0.012502 0.026393 0.026393 0.026393 0.026393
  spline S19 degree 3 poles (-15.4217, -5.2904) (-15.4191, -5.336) (-15.4143, -5.4246) (-15.3732, -5.5032) (-15.3533, -5.5414) knots 0 0 0 0 0.013512 0.026281 0.026281 0.026281 0.026281
  spline S20 degree 3 poles (-15.3533, -5.5414) (-15.3278, -5.5747) (-15.2764, -5.6421) (-15.1977, -5.6738) (-15.158, -5.6898) knots 0 0 0 0 0.01234 0.02494 0.02494 0.02494 0.02494
  spline S21 degree 3 poles (-15.158, -5.6898) (-15.1007, -5.7014) (-14.9572, -5.7304) (-14.8105, -5.73) (-14.7224, -5.7299) knots 0 0 0 0 0.017496 0.043833 0.043833 0.043833 0.043833
  line L12 (-20.8982, -5.7299) -> (-20.1658, -5.7299)
  line L13 (-20.1658, -5.7299) -> (-20.1658, -4.7064)
  line L14 (-20.1658, -4.7064) -> (-20.906, -4.7064)
  spline S22 degree 3 poles (-20.906, -4.7064) (-21.0136, -4.7076) (-21.2001, -4.7098) (-21.3599, -4.8035) (-21.4275, -4.8431) knots 0 0 0 0 0.031582 0.054729 0.054729 0.054729 0.054729
  spline S23 degree 3 poles (-21.4275, -4.8431) (-21.4725, -4.8953) (-21.5674, -5.0055) (-21.5768, -5.1512) (-21.5818, -5.2279) knots 0 0 0 0 0.020117 0.042474 0.042474 0.042474 0.042474
  spline S24 degree 3 poles (-21.5818, -5.2279) (-21.5786, -5.2848) (-21.5724, -5.3946) (-21.5175, -5.4897) (-21.491, -5.5355) knots 0 0 0 0 0.016829 0.032476 0.032476 0.032476 0.032476
  spline S25 degree 3 poles (-21.491, -5.5355) (-21.4584, -5.5745) (-21.3937, -5.6521) (-21.2989, -5.6871) (-21.2517, -5.7045) knots 0 0 0 0 0.01495 0.029749 0.029749 0.029749 0.029749
  spline S26 degree 3 poles (-21.2517, -5.7045) (-21.2064, -5.7118) (-21.0894, -5.7307) (-20.9708, -5.7302) (-20.8982, -5.7299) knots 0 0 0 0 0.013756 0.035493 0.035493 0.035493 0.035493
  spline S27 degree 3 poles (-58.0341, -14.4706) (-57.9047, -14.4591) (-57.6462, -14.4362) (-57.4431, -14.2748) (-57.3417, -14.1942) knots 0 0 0 0 0.038059 0.076028 0.076028 0.076028 0.076028
  spline S28 degree 3 poles (-57.3417, -14.1942) (-57.2575, -14.0753) (-57.0634, -13.8012) (-57.0559, -13.4629) (-57.0516, -13.2713) knots 0 0 0 0 0.042826 0.098694 0.098694 0.098694 0.098694
  spline S29 degree 3 poles (-57.0516, -13.2713) (-57.0599, -13.1118) (-57.0753, -12.8125) (-57.2489, -12.5694) (-57.33, -12.4559) knots 0 0 0 0 0.046785 0.087776 0.087776 0.087776 0.087776
  spline S30 degree 3 poles (-57.33, -12.4559) (-57.4292, -12.369) (-57.6294, -12.1938) (-57.8945, -12.17) (-58.0282, -12.1581) knots 0 0 0 0 0.038513 0.077679 0.077679 0.077679 0.077679
  spline S31 degree 3 poles (-58.0282, -12.1581) (-58.1639, -12.1699) (-58.4316, -12.1933) (-58.633, -12.3711) (-58.7323, -12.4588) knots 0 0 0 0 0.039708 0.078388 0.078388 0.078388 0.078388
  spline S32 degree 3 poles (-58.7323, -12.4588) (-58.8128, -12.5762) (-58.9883, -12.8323) (-59.0015, -13.1437) (-59.0087, -13.3124) knots 0 0 0 0 0.041868 0.091327 0.091327 0.091327 0.091327
  spline S33 degree 3 poles (-59.0087, -13.3124) (-59.0049, -13.4227) (-58.9976, -13.6325) (-58.925, -13.8294) (-58.8905, -13.9227) knots 0 0 0 0 0.032872 0.062524 0.062524 0.062524 0.062524
  spline S34 degree 3 poles (-58.8905, -13.9227) (-58.8472, -14.0043) (-58.762, -14.1649) (-58.6164, -14.2736) (-58.5448, -14.327) knots 0 0 0 0 0.027339 0.053788 0.053788 0.053788 0.053788
  spline S35 degree 3 poles (-58.5448, -14.327) (-58.466, -14.3689) (-58.3063, -14.4538) (-58.1256, -14.4649) (-58.0341, -14.4706) knots 0 0 0 0 0.026437 0.053604 0.053604 0.053604 0.053604
  spline S36 degree 3 poles (-48.6634, -14.5215) (-48.534, -14.51) (-48.2756, -14.4871) (-48.0725, -14.3257) (-47.971, -14.2451) knots 0 0 0 0 0.038059 0.076028 0.076028 0.076028 0.076028
  spline S37 degree 3 poles (-47.971, -14.2451) (-47.8868, -14.1262) (-47.6927, -13.8521) (-47.6852, -13.5138) (-47.681, -13.3223) knots 0 0 0 0 0.042826 0.098694 0.098694 0.098694 0.098694
  spline S38 degree 3 poles (-47.681, -13.3223) (-47.6892, -13.1627) (-47.7046, -12.8634) (-47.8782, -12.6204) (-47.9593, -12.5069) knots 0 0 0 0 0.046785 0.087776 0.087776 0.087776 0.087776
  spline S39 degree 3 poles (-47.9593, -12.5069) (-48.0586, -12.42) (-48.2588, -12.2448) (-48.5239, -12.221) (-48.6576, -12.209) knots 0 0 0 0 0.038513 0.077679 0.077679 0.077679 0.077679
  spline S40 degree 3 poles (-48.6576, -12.209) (-48.7932, -12.2209) (-49.061, -12.2443) (-49.2623, -12.4221) (-49.3617, -12.5098) knots 0 0 0 0 0.039708 0.078388 0.078388 0.078388 0.078388
  spline S41 degree 3 poles (-49.3617, -12.5098) (-49.4421, -12.6272) (-49.6176, -12.8832) (-49.6309, -13.1946) (-49.638, -13.3633) knots 0 0 0 0 0.041868 0.091327 0.091327 0.091327 0.091327
  spline S42 degree 3 poles (-49.638, -13.3633) (-49.6342, -13.4736) (-49.6269, -13.6835) (-49.5543, -13.8803) (-49.5199, -13.9737) knots 0 0 0 0 0.032872 0.062524 0.062524 0.062524 0.062524
  spline S43 degree 3 poles (-49.5199, -13.9737) (-49.4766, -14.0553) (-49.3914, -14.2159) (-49.2458, -14.3245) (-49.1742, -14.3779) knots 0 0 0 0 0.027339 0.053788 0.053788 0.053788 0.053788
  spline S44 degree 3 poles (-49.1742, -14.3779) (-49.0954, -14.4198) (-48.9356, -14.5047) (-48.755, -14.5159) (-48.6634, -14.5215) knots 0 0 0 0 0.026437 0.053604 0.053604 0.053604 0.053604
  spline S45 degree 3 poles (-25.4685, -4.6049) (-25.3899, -4.5986) (-25.2358, -4.5863) (-25.1161, -4.4886) (-25.0574, -4.4408) knots 0 0 0 0 0.023049 0.045211 0.045211 0.045211 0.045211
  spline S46 degree 3 poles (-25.0574, -4.4408) (-25.0098, -4.382) (-24.913, -4.2623) (-24.9006, -4.1088) (-24.8943, -4.0306) knots 0 0 0 0 0.022142 0.045066 0.045066 0.045066 0.045066
  spline S47 degree 3 poles (-24.8943, -4.0306) (-24.8974, -3.9806) (-24.9037, -3.8794) (-24.9448, -3.7866) (-24.9656, -3.7396) knots 0 0 0 0 0.014902 0.030175 0.030175 0.030175 0.030175
  spline S48 degree 3 poles (-24.9656, -3.7396) (-24.9924, -3.6953) (-25.0461, -3.6064) (-25.1336, -3.5501) (-25.1775, -3.5219) knots 0 0 0 0 0.015303 0.030747 0.030747 0.030747 0.030747
  spline S49 degree 3 poles (-25.1775, -3.5219) (-25.2254, -3.4994) (-25.3213, -3.4542) (-25.4272, -3.4479) (-25.4802, -3.4447) knots 0 0 0 0 0.015704 0.031496 0.031496 0.031496 0.031496
  spline S50 degree 3 poles (-25.4802, -3.4447) (-25.5599, -3.4508) (-25.7152, -3.4626) (-25.8369, -3.5595) (-25.8963, -3.6068) knots 0 0 0 0 0.023352 0.045577 0.045577 0.045577 0.045577
  spline S51 degree 3 poles (-25.8963, -3.6068) (-25.9441, -3.6654) (-26.042, -3.7853) (-26.0541, -3.9399) (-26.0603, -4.0189) knots 0 0 0 0 0.022142 0.045311 0.045311 0.045311 0.045311
  spline S52 degree 3 poles (-26.0603, -4.0189) (-26.0539, -4.0993) (-26.0412, -4.2571) (-25.9406, -4.379) (-25.8914, -4.4388) knots 0 0 0 0 0.023575 0.046245 0.046245 0.046245 0.046245
  spline S53 degree 3 poles (-25.8914, -4.4388) (-25.8307, -4.4873) (-25.707, -4.586) (-25.5491, -4.5985) (-25.4685, -4.6049) knots 0 0 0 0 0.022732 0.046366 0.046366 0.046366 0.046366
  spline S54 degree 3 poles (-25.4744, -5.7904) (-25.4107, -5.7856) (-25.2863, -5.7761) (-25.1883, -5.6991) (-25.1404, -5.6615) knots 0 0 0 0 0.018688 0.036526 0.036526 0.036526 0.036526
  spline S55 degree 3 poles (-25.1404, -5.6615) (-25.1017, -5.6167) (-25.0248, -5.5278) (-25.0133, -5.4109) (-25.0076, -5.3529) knots 0 0 0 0 0.017313 0.034339 0.034339 0.034339 0.034339
  spline S56 degree 3 poles (-25.0076, -5.3529) (-25.0124, -5.2889) (-25.0218, -5.1645) (-25.1003, -5.0678) (-25.1384, -5.0209) knots 0 0 0 0 0.018745 0.036458 0.036458 0.036458 0.036458
  spline S57 degree 3 poles (-25.1384, -5.0209) (-25.1865, -4.9833) (-25.2862, -4.9053) (-25.4127, -4.8965) (-25.4783, -4.892) knots 0 0 0 0 0.017879 0.037096 0.037096 0.037096 0.037096
  spline S58 degree 3 poles (-25.4783, -4.892) (-25.5422, -4.8966) (-25.6664, -4.9057) (-25.764, -4.9826) (-25.8113, -5.0199) knots 0 0 0 0 0.018756 0.03641 0.03641 0.03641 0.03641
  spline S59 degree 3 poles (-25.8113, -5.0199) (-25.8492, -5.0651) (-25.9253, -5.1559) (-25.9359, -5.274) (-25.9412, -5.3334) knots 0 0 0 0 0.017248 0.034667 0.034667 0.034667 0.034667
  spline S60 degree 3 poles (-25.9412, -5.3334) (-25.9358, -5.3951) (-25.9251, -5.5175) (-25.8464, -5.6118) (-25.8074, -5.6586) knots 0 0 0 0 0.018109 0.035925 0.035925 0.035925 0.035925
  spline S61 degree 3 poles (-25.8074, -5.6586) (-25.7595, -5.697) (-25.6622, -5.7752) (-25.5377, -5.7853) (-25.4744, -5.7904) knots 0 0 0 0 0.017978 0.036559 0.036559 0.036559 0.036559
  point P0 (-13.5107, -16.398)
  point P1 (-13, -12)
  point P2 (-13.8677, -6.5042)
  point P3 (-16.4431, -4.6361)
  point P4 (-22.9998, -4.2631)
  point P5 (-26.866, -5.434)
  point P6 (-29.8813, -5.3314)
  point P7 (-30.6463, -7.6772)
  point P8 (-32, -6)
  point P9 (-35.5422, -4.0563)
  point P10 (-40.4381, -3.5973)
  point P11 (-44, -4)
  point P12 (-45, -4)
  point P13 (-53, -4)
  point P14 (-58.7662, -3.649)
  point P15 (-59.7, -6.5)
  point P16 (-59.7, -11.1451)
  point P17 (-59.1036, -13.1835)
  point P18 (-56.8251, -12.5624)
  point P19 (-51.5134, -13.8825)
  point P20 (-47.4759, -13.2772)
  point P21 (-45.4869, -16.704)
  point P22 (-42, -19)
  point P23 (-38, -20)
  point P24 (-34, -19)
  point P25 (-32.1763, -16.449)
  point P26 (-30.6973, -13.3393)
  point P27 (-28.6573, -13.0366)
  point P28 (-23.4555, -13.3393)
  point P29 (-18.9166, -14.4223)
  point P30 (-22.0785, -16.5)
  point P31 (-24, -21)
  point P32 (-19.85, -21.05)
  point P33 (-14.3267, -21.05)
  point P34 (-17.5906, -21.7019)
split "Split1" [suppressed]
sketch "Sketch22" plane through (0, 0, 9.1) normal (0, 0, 1) x (-1, 0, 0)
  line L0 (-13.9, -12.5) -> (-16.45, -12.5)
  line L1 (-16.45, -12.5) -> (-16.45, -16.5)
  line L2 (-16.45, -16.5) -> (-13.9, -16.5)
  line L3 (-13.9, -16.5) -> (-13.9, -12.5)
  line L4 (-13.9, -12.5) -> (-15.65, -12.5)
  line L5 (-15.65, -12.5) -> (-15.65, -16.5)
  line L6 (-15.65, -16.5) -> (-13.9, -16.5)
  line L7 (-13.9, -16.5) -> (-13.9, -12.5)
  dimension "d165" = 1.75
  dimension "d166" = 4
  constraint horizontal L4
  constraint vertical L5
  constraint horizontal L6
  constraint vertical L7
  constraint coincident L0.start L3.end
  measures "d165" distance of L0.start L4.end
  measures "d166" distance of L0.start L2.end
extrude "Extrude26" add sketch "Sketch22" along normal blind 1 contours L0 L2 L3 L4 L5 L6 L7 bodies 1
fillet "Fillet3" radius 0.5 1 edges at (15.65, 14.5, 9.1) on bodies 1
equation "d13 = ( d1 - d12 ) / 2"
equation "d15 = ( d2 - d14 ) / 2"
equation "d48 = ( 25.00 mm - ( 4 * 4 ) * 1 mm ) / 2"
equation "d55 = ( 25.00 mm - ( 4 * 4 ) * 1 mm ) / 2"
equation "d64 = ( 69.40 mm - ( 15 * 4 ) * 1 mm ) / 2"
equation "d108 = 3.5 mm + 1.6 mm"
equation "d118 = ( 66.40 mm - d115 ) / 2"
equation "d123 = ( 66.40 mm - d120 ) / 2"
